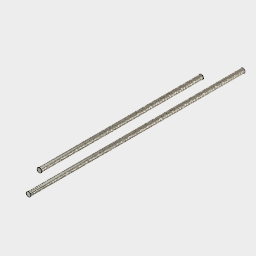
X_Axis_v8 (Autodesk Fusion 360 archive; units mm, degrees)
design "Z Linear Rods"
Autodesk Fusion 360 part; units mm, degrees
note: some values were not read from the file. Chosen so that the rebuilt part matches the saved one: how an offset face is resized.
sketch "Sketch1" plane through (0, 0, 0) normal (0, 1, 0) x (1, 0, 0) in component "X Linear Rods"
  circle A0 centre (0, 0) radius 3
  dimension "d1" = 6
  measures "d1" diameter of A0
extrude "Extrude1" add sketch "Sketch1" along normal mid plane 210 makes body 1 in component "Short"
extrude "Extrude1'" add sketch "Sketch1" along normal mid plane 278 separate body makes body 2 in component "Long"
component "X Linear Rods" placed x (1, 0, 0) y (0, 1, 0) z (0, 0, 1) at (0, 0, 0)
component "Short" placed x (1, 0, 0) y (0, 1, 0) z (0, 0, 1) at (-20, 0, 0) in component "X Linear Rods"
component "Long" placed x (1, 0, 0) y (0, 1, 0) z (0, 0, 1) at (0, 0, 0) in component "X Linear Rods"

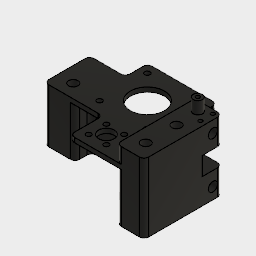
design "Z Carriage"
Autodesk Fusion 360 part; units mm, degrees
sketch "Base" plane through (0, 0, 0) normal (0, 0, 1) x (1, 0, 0) in component "Z Carriage"
  line L0 (-43.6, -8.8) -> (-23.6, -8.8)
  line L1 (-23.6, -8.8) -> (-23.6, 20.7)
  line L2 (-23.6, 20.7) -> (-43.6, 20.7)
  line L3 (-43.6, 20.7) -> (-43.6, -8.8)
  line L4 (-23.6, 2) -> (24.6, 2)
  line L5 (24.6, 2) -> (24.6, 5.65)
  line L6 (24.6, 5.65) -> (-23.6, 5.65)
  line L7 (-23.6, 5.65) -> (-23.6, 2)
  line L8 (24.6, 20.7) -> (42.4, 20.7)
  line L9 (42.4, 20.7) -> (42.4, -30)
  line L10 (42.4, -30) -> (24.6, -30)
  line L11 (24.6, -30) -> (24.6, 20.7)
  line L12 (35.44, 20.7) -> (35.44, 14.8) construction
  line L13 (38.78, 20.7) -> (38.78, 18.14)
  line L14 (32.1, 20.7) -> (32.1, 18.14)
  line L15 (32.1, 18.14) -> (38.78, 18.14) construction
  arc A0 (32.1, 18.14) -> (38.78, 18.14) centre (35.44, 18.14) ccw
  circle A1 centre (35.44, 18.14) radius 1.25
  circle A2 centre (-33.5, 0) radius 6
  circle A3 centre (-33.5, 0) radius 3
  circle A4 centre (33.5, 0) radius 3
  circle A5 centre (33.5, 0) radius 6
  circle A6 centre (33.5, -20) radius 6
  circle A7 centre (33.5, -20) radius 3
  line L16 (33.5, -20) -> (33.5, 0) construction
  line L17 (33.5, 0) -> (-33.5, 0) construction
  line L18 (33.5, -30) -> (33.5, -20) construction
  point P0 (35.44, 18.14)
  point P1 (33.5, -26)
  dimension "d1" = 48.2
  dimension "d2" = 20
  dimension "d3" = 17.8
  dimension "d4" = 3.65
  dimension "d5" = 29.5
  dimension "d6" = 50.7
  dimension "d8" = 32
  dimension "d9" = 5.9
  dimension "d11" = 6.68
  dimension "d12" = 7.5
  dimension "d13" = 2.5
  dimension "d14" = 12
  dimension "d15" = 6
  dimension "d16" = 6
  dimension "d17" = 12
  dimension "d18" = 12
  dimension "d19" = 6
  dimension "d20" = 67
  dimension "d21" = 20
  dimension "d23" = 4
  measures "d1" distance of L5.end L6.end
  measures "d2" distance of L1.end L2.end
  measures "d3" distance of L8.start L8.end
  measures "d4" distance of L4 L6
  measures "d5" distance of L0.start L2.end
  measures "d6" distance of L8.end L9.end
  measures "d8" distance of L4 L10.end
  measures "d9" distance of L12.start L12.end
  measures "d11" distance of L13.start L14.start
  measures "d12" distance of L8.start L14.start
  measures "d13" diameter of A1
  measures "d14" diameter of A2
  measures "d15" diameter of A3
  measures "d16" diameter of A4
  measures "d17" diameter of A5
  measures "d18" diameter of A6
  measures "d19" diameter of A7
  measures "d20" distance of A4.centre A2.centre
  measures "d21" distance of A6.centre A4.centre
  measures "d23" distance of L18.start P1
extrude "Extrude1" add sketch "Base" along normal blind 35 contours L0 L1 L2 L3 L7 | L1 L4 L5 L6 L7 L11 | A2 in component "Z Carriage"
extrude "Extrude2" add sketch "Base" along normal blind 45 contours L5 L8 L9 L10 L11 L13 L14 A0 | L8 L13 L14 A0 | A1 | A5 | A6 in component "Z Carriage"
extrude "Extrude3" add sketch "Base" against normal blind 3 contours L8 L13 L14 A0 in component "Z Carriage"
fillet "Fillet1" radius 3 12 edges at (24.6, 2, 17.5) (24.6, 5.65, 17.5) (-23.6, 2, 17.5) (-23.6, 5.65, 17.5) (-23.6, 20.7, 17.5) (-43.6, 20.7, 17.5) (-43.6, -8.8, 17.5) (-23.6, -8.8, 17.5) (24.6, 20.7, 22.5) (42.4, 20.7, 22.5) (42.4, -30, 22.5) (24.6, -30, 22.5) in component "Z Carriage"
sketch "Top Endstop Mount" plane through (0, 0, 35) normal (0, 0, 1) x (-1, 0, 0) in component "Z Carriage"
  line L0 (26.6, -20.7) -> (20.4, -20.7)
  line L1 (20.4, -20.7) -> (20.4, -35.1993)
  line L2 (20.4, -35.1993) -> (-24.6, -35.1993)
  line L3 (-24.6, -35.1993) -> (-24.6, -17.7)
  line L4 (-27.6, 30) -> (-39.4, 30)
  line L5 (26.6, -20.7) -> (40.6, -20.7)
  arc A0 (40.6, -20.7) -> (43.6, -17.7) centre (40.6, -17.7) ccw
  line L6 (43.6, -17.7) -> (43.6, 5.8)
  arc A1 (43.6, 5.8) -> (40.6, 8.8) centre (40.6, 5.8) ccw
  line L7 (40.6, 8.8) -> (26.6, 8.8)
  arc A2 (-24.6, 27) -> (-27.6, 30) centre (-27.6, 27) ccw
  line L8 (-24.6, -17.7) -> (-24.6, 27)
  line L9 (-27.6, 30) -> (5.6, 30)
  line L10 (5.6, 30) -> (5.6, 8.8)
  line L11 (5.6, 8.8) -> (26.6, 8.8)
  arc A3 (-39.4, 30) -> (-42.4, 27) centre (-39.4, 27) ccw
  line L12 (-42.4, 27) -> (-42.4, -17.7)
  arc A4 (-42.4, -17.7) -> (-39.4, -20.7) centre (-39.4, -17.7) ccw
  line L13 (-39.4, -20.7) -> (-27.6, -20.7)
  arc A5 (-27.6, -20.7) -> (-24.6, -17.7) centre (-27.6, -17.7) ccw
  line L14 (15.1, -29.6993) -> (-15.9, -29.6993) construction
  line L15 (-15.9, -29.6993) -> (-15.9, 1.3007) construction
  line L16 (-15.9, 1.3007) -> (15.1, 1.3007) construction
  line L17 (15.1, 1.3007) -> (15.1, -29.6993) construction
  line L18 (15.1, 1.3007) -> (-15.9, -29.6993) construction
  circle A6 centre (-0.4, -14.1993) radius 11
  circle A7 centre (15.1, -29.6993) radius 1.725
  circle A8 centre (-15.9, -29.6993) radius 1.725
  circle A9 centre (-15.9, 1.3007) radius 1.725
  circle A10 centre (15.1, 1.3007) radius 1.725
  line L19 (-0.25, 12.25) -> (-11.75, 12.25) construction
  line L20 (-11.75, 12.25) -> (-11.75, 23.75) construction
  line L21 (-11.75, 23.75) -> (-0.25, 23.75) construction
  line L22 (-0.25, 23.75) -> (-0.25, 12.25) construction
  circle A11 centre (-11.75, 12.25) radius 1.65
  circle A12 centre (-11.75, 23.75) radius 1.65
  circle A13 centre (-0.25, 23.75) radius 1.65
  circle A14 centre (-0.25, 12.25) radius 1.65
  line L23 (-0.25, 23.75) -> (-11.75, 12.25) construction
  circle A15 centre (-6, 18) radius 5
  line L24 (-27.6, -20.7) -> (-24.6, -20.7)
  circle A16 centre (33.5, 0) radius 3
  circle A17 centre (33.5, 0) radius 3
  circle A18 centre (-33.5, 20) radius 3
  point P0 (-24.6, -17.7)
  point P1 (20.6, -5.65)
  dimension "d31" = 48
  dimension "d32" = 45
  dimension "d33" = 29.55
  dimension "d34" = 31
  dimension "d35" = 31
  dimension "d36" = 22
  dimension "d37" = 44
  dimension "d38" = 3.45
  dimension "d39" = 3.45
  dimension "d40" = 3.45
  dimension "d41" = 3.45
  dimension "d42" = 21
  dimension "d43" = 11.5
  dimension "d44" = 11.5
  dimension "d45" = 3.3
  dimension "d46" = 3.3
  dimension "d47" = 3.3
  dimension "d48" = 3.3
  dimension "d49" = 10
  dimension "d85" = 27.5
  dimension "d86" = 2
  measures "d31" distance of L9.end A3.end
  measures "d32" distance of L1.end L2.end
  measures "d33" distance of L1.end P1
  measures "d34" distance of L14.start L14.end
  measures "d35" distance of L14.start L16.end
  measures "d36" diameter of A6
  measures "d37" distance of L6 A6.centre
  measures "d38" diameter of A7
  measures "d39" diameter of A8
  measures "d40" diameter of A9
  measures "d41" diameter of A10
  measures "d42" distance of L2 A6.centre
  measures "d43" distance of L19.start L19.end
  measures "d44" distance of L19.start L21.end
  measures "d45" diameter of A11
  measures "d46" diameter of A12
  measures "d47" diameter of A13
  measures "d48" diameter of A14
  measures "d49" diameter of A15
  measures "d85" distance of A15.centre A18.centre
  measures "d86" distance of A15.centre A18.centre
extrude "Extrude4" add sketch "Top Endstop Mount" against normal blind 3 contours L0 L1 L2 L3 L5 A0 L6 A1 L7 A2 L8 L9 L10 L11 | L3 A5 L24 in component "Z Carriage"
extrude "Extrude10" cut sketch "Top Endstop Mount" against normal blind 3 contours A6 in component "Z Carriage"
extrude "Extrude7" add sketch "Top Endstop Mount" along normal blind 10 contours L3 A5 L24 in component "Z Carriage"
fillet "Fillet2" radius 3 5 edges at (-20.4, 35.1993, 33.5) (-20.4, 20.7, 33.5) (-5.6, -8.8, 33.5) (-5.6, -30, 33.5) (24.6, 35.1993, 33.5) in component "Z Carriage"
sketch "Face" plane through (42.4, 0, 0) normal (1, 0, 0) x (0, 1, 0) in component "Z Carriage"
  line L0 (14.7, 37.5) -> (14.7, 7.5) construction
  circle A0 centre (14.7, 37.5) radius 3
  circle A1 centre (14.7, 7.5) radius 3
  line L1 (20.7, 0) -> (20.7, 45)
  line L2 (20.7, 22.5) -> (14.7, 22.5) construction
  line L3 (20.7, 28.4) -> (7.73, 28.4)
  line L4 (7.73, 28.4) -> (7.73, 16.6)
  line L5 (7.73, 16.6) -> (20.7, 16.6)
  point P0 (7.73, 22.5)
  dimension "d55" = 6
  dimension "d56" = 6
  dimension "d58" = 30
  dimension "d59" = 6
  dimension "d64" = 12.97
  dimension "d65" = 11.8
  measures "d55" diameter of A0
  measures "d56" diameter of A1
  measures "d58" distance of L0.start L0.end
  measures "d59" distance of L2.start L2.end
  measures "d64" distance of L3.start L3.end
  measures "d65" distance of L3.end L4.end
extrude "Extrude5" cut sketch "Face" against normal blind 17.81 contours A0 | L1 L3 L4 L5 in component "Z Carriage"
extrude "Extrude6" cut sketch "Face" against normal blind 86 contours A1 in component "Z Carriage"
sketch "Top Mount" plane through (0, 0, 45) normal (0, 0, 1) x (-1, 0, 0) in component "Z Carriage"
  arc A0 (-24.6, 27) -> (-27.6, 30) centre (-27.6, 27) ccw
  line L0 (-27.6, 30) -> (-39.4, 30)
  arc A1 (-39.4, 30) -> (-42.4, 27) centre (-39.4, 27) ccw
  line L1 (-42.4, 27) -> (-42.4, -17.7)
  arc A2 (-42.4, -17.7) -> (-39.4, -20.7) centre (-39.4, -17.7) ccw
  line L2 (-39.4, -20.7) -> (-24.6, -20.7)
  line L3 (-27.6, -20.7) -> (-24.6, -20.7)
  line L4 (-39.4, -20.7) -> (-27.6, -20.7)
  arc A3 (-42.4, -17.7) -> (-39.4, -20.7) centre (-39.4, -17.7) ccw
  line L5 (-42.4, 27) -> (-42.4, -17.7)
  arc A4 (-24.6, 27) -> (-27.6, 30) centre (-27.6, 27) ccw
  line L6 (-27.6, 30) -> (-39.4, 30)
  arc A5 (-39.4, 30) -> (-42.4, 27) centre (-39.4, 27) ccw
  line L7 (-24.6, -20.7) -> (-24.6, 27)
  circle A6 centre (-32.6, -14.7) radius 3
  circle A7 centre (-32.6, -14.7) radius 1.25
  line L8 (-38.95, -18.07) -> (-38.95, -10.07)
  circle A8 centre (-38.95, -18.07) radius 1.25
  circle A9 centre (-38.95, -10.07) radius 1.25
  circle A10 centre (-33.5, 20) radius 3
  circle A11 centre (-33.5, 0) radius 3
  circle A12 centre (-33.5, 0) radius 3
  circle A13 centre (-33.5, 20) radius 3
  dimension "d70" = 6
  dimension "d71" = 2.5
  dimension "d72" = 6
  dimension "d73" = 8
  dimension "d74" = 2.5
  dimension "d75" = 2.5
  dimension "d76" = 8
  dimension "d77" = 2.63
  dimension "d78" = 3.45
  measures "d70" diameter of A6
  measures "d71" diameter of A7
  measures "d72" distance of L2.end A6.centre
  measures "d73" distance of L2.end A6.centre
  measures "d74" diameter of A8
  measures "d75" diameter of A9
  measures "d76" distance of L8.start L8.end
  measures "d77" distance of A2.end L8.start
  measures "d78" distance of L1.end L8.start
extrude "Extrude8" add sketch "Top Mount" along normal blind 8 contours A6 in component "Z Carriage"
extrude "Extrude9" cut sketch "Top Mount" against normal blind 5 contours A8 | A9 in component "Z Carriage"
component "Z Carriage" placed x (1, 0, 0) y (0, 1, 0) z (0, 0, 1) at (0, 0, 0)
equation "d77 = 1.38 mm + d74 / 2"
equation "d78 = 2.2 mm + d74 / 2"

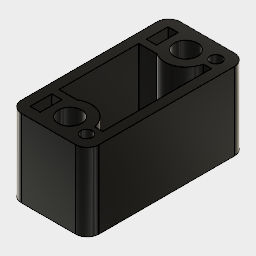
design "X End Bracket"
Autodesk Fusion 360 part; units mm, degrees
sketch "Outside" plane through (0, 0, 0) normal (0, 0, 1) x (1, 0, 0) in component "X End Bracket"
  line L0 (10, -20.5) -> (-10, -20.5)
  line L1 (-10, -20.5) -> (-10, 20.5)
  line L2 (-10, 20.5) -> (10, 20.5)
  line L3 (10, 20.5) -> (10, -20.5)
  line L4 (0, -20.5) -> (0, 20.5) construction
  circle A0 centre (0, 0) radius 2.95
  circle A1 centre (0, 0) radius 1.6
  circle A2 centre (0, 14.965) radius 3
  circle A3 centre (0, 14.965) radius 1.575
  line L5 (10, 0) -> (-10, 0) construction
  line L6 (6, 16.7) -> (6, -16.7)
  circle A4 centre (6, 16.7) radius 1.5
  circle A5 centre (6, -16.7) radius 1.5
  circle A6 centre (0, -14.965) radius 3
  circle A7 centre (0, -14.965) radius 1.575
  circle A8 centre (0, 0) radius 5
  point P0 (6, 0)
  dimension "d1" = 20
  dimension "d2" = 41
  dimension "d3" = 5.9
  dimension "d4" = 3.2
  dimension "d5" = 6
  dimension "d6" = 3.15
  dimension "d8" = 14.965
  dimension "d9" = 3
  dimension "d10" = 3
  dimension "d11" = 33.4
  dimension "d12" = 4
  dimension "d32" = 10
  measures "d1" distance of L0.start L0.end
  measures "d2" distance of L0.start L2.end
  measures "d3" diameter of A0
  measures "d4" diameter of A1
  measures "d5" diameter of A2
  measures "d6" diameter of A3
  measures "d8" distance of A2.centre L5.end
  measures "d9" diameter of A4
  measures "d10" diameter of A5
  measures "d11" distance of L6.start L6.end
  measures "d12" distance of L3 L6
  measures "d32" diameter of A8
extrude "Extrude1" add sketch "Outside" along normal blind 20 contours L0 L1 L2 L3 | A0 | A8 in component "X End Bracket"
extrude "Extrude2" add sketch "Outside" along normal blind 1.88 contours A2 | A6 in component "X End Bracket"
extrude "Extrude3" cut sketch "Outside" along normal blind 3 contours A0 in component "X End Bracket"
fillet "Fillet1" radius 3 4 edges at (10, 20.5, 10) (-10, 20.5, 10) (-10, -20.5, 10) (10, -20.5, 10) in component "X End Bracket"
sketch "Inside" plane through (0, 0, 20) normal (0, 0, 1) x (-1, 0, 0) in component "X End Bracket"
  circle A0 centre (0, 14.965) radius 3
  circle A1 centre (-6, -16.7) radius 1.5
  circle A2 centre (-6, 16.7) radius 1.5
  circle A3 centre (0, -14.965) radius 3 construction
  arc A4 (-7, 20.5) -> (-10, 17.5) centre (-7, 17.5) ccw
  line L0 (-10, 17.5) -> (-10, -17.5)
  arc A5 (-10, -17.5) -> (-7, -20.5) centre (-7, -17.5) ccw
  line L1 (-7, -20.5) -> (7, -20.5)
  arc A6 (7, -20.5) -> (10, -17.5) centre (7, -17.5) ccw
  line L2 (10, -17.5) -> (10, 17.5)
  arc A7 (10, 17.5) -> (7, 20.5) centre (7, 17.5) ccw
  line L3 (7, 20.5) -> (-7, 20.5)
  line L4 (-10, 0) -> (10, 0) construction
  line L5 (0, -20.5) -> (0, 20.5) construction
  line L6 (-10, 17.5) -> (-10, -17.5)
  arc A8 (-10, -17.5) -> (-7, -20.5) centre (-7, -17.5) ccw
  line L7 (-7, -20.5) -> (7, -20.5)
  arc A9 (7, -20.5) -> (10, -17.5) centre (7, -17.5) ccw
  line L8 (10, -17.5) -> (10, 17.5)
  arc A10 (10, 17.5) -> (7, 20.5) centre (7, 17.5) ccw
  line L9 (7, 20.5) -> (-7, 20.5)
  arc A11 (-7, 20.5) -> (-10, 17.5) centre (-7, 17.5) ccw
  line L10 (-10, -17.5) -> (-10, 17.5)
  circle A12 centre (-6, -16.7) radius 1.5
  circle A13 centre (0, -14.965) radius 3
  circle A14 centre (0, 14.965) radius 3
  circle A15 centre (-6, 16.7) radius 1.5
  circle A16 centre (0, -14.965) radius 5.5 construction
  line L11 (10, -10.3) -> (2.9134, -10.3)
  line L12 (-10, -14) -> (-5.4147, -14)
  line L13 (7.45, -17.8) -> (4.85, -17.8)
  line L14 (4.85, -17.8) -> (4.85, -12.2)
  line L15 (4.85, -12.2) -> (7.45, -12.2)
  line L16 (7.45, -12.2) -> (7.45, -17.8)
  arc A17 (2.9134, -10.3) -> (-5.4147, -14) centre (0, -14.965) ccw
  line L17 (4.85, 17.8) -> (4.85, 12.2)
  line L18 (4.85, 12.2) -> (7.45, 12.2)
  line L19 (7.45, 17.8) -> (4.85, 17.8)
  line L20 (7.45, 12.2) -> (7.45, 17.8)
  line L21 (10, 10.3) -> (2.9134, 10.3)
  arc A18 (-5.4147, 14) -> (2.9134, 10.3) centre (0, 14.965) ccw
  line L22 (-10, 14) -> (-5.4147, 14)
  line L23 (7.5, -10.3) -> (7.5, 10.3)
  line L24 (-7.5, -14) -> (-7.5, 14)
  dimension "d20" = 11
  dimension "d22" = 10.3
  dimension "d23" = 14
  dimension "d24" = 5.6
  dimension "d25" = 1.9
  dimension "d26" = 2.55
  dimension "d27" = 2.6
  dimension "d28" = 2.5
  dimension "d29" = 2.5
  measures "d20" diameter of A16
  measures "d22" distance of L4.end L11
  measures "d23" distance of L4.start L12
  measures "d24" distance of L13.start L15.end
  measures "d25" distance of L11.start L15.end
  measures "d26" distance of A6.end L13.start
  measures "d27" distance of L13.start L13.end
  measures "d28" distance of L2 L23
  measures "d29" distance of L0 L24
extrude "Extrude4" cut sketch "Inside" against normal blind 17 contours L11 L12 A17 L21 A18 L22 L23 L24 | L13 L14 L15 L16 | L17 L18 L19 L20 in component "X End Bracket"
extrude "Extrude5" add sketch "Outside" along normal blind 1.5 from surface at 3 contours A0 | A8 in component "X End Bracket"
component "X End Bracket" placed x (1, 0, 0) y (0, 1, 0) z (0, 0, 1) at (0, 0, 0)
equation "d8 = ( 29.93 / 2 ) * 1 mm"
equation "d22 = ( 20.6 / 2 ) * 1 mm"
equation "d23 = ( 28 / 2 ) * 1 mm"

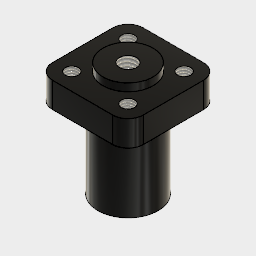
design "Lead Srew Nut"
Autodesk Fusion 360 part; units mm, degrees
sketch "Sketch1" plane through (0, 0, 0) normal (0, 0, 1) x (1, 0, 0) in component "Lead Srew Nut"
  circle A0 centre (0, 0) radius 4.9
  circle A1 centre (0, 0) radius 5.9
  circle A2 centre (0, 0) radius 2
  line L0 (-5.9, 8.9) -> (5.9, 8.9)
  line L1 (8.9, 5.9) -> (8.9, -5.9)
  line L2 (5.9, -8.9) -> (-5.9, -8.9)
  line L3 (-8.9, -5.9) -> (-8.9, 5.9)
  line L4 (-8.9, 8.9) -> (8.9, -8.9) construction
  line L5 (8.9, 8.9) -> (-8.9, -8.9) construction
  circle A3 centre (-5.5, 5.5) radius 1.5
  circle A4 centre (-5.5, -5.5) radius 1.5
  circle A5 centre (5.5, -5.5) radius 1.5
  circle A6 centre (5.5, 5.5) radius 1.5
  arc A7 (-5.9, 8.9) -> (-8.9, 5.9) centre (-5.9, 5.9) ccw
  arc A8 (8.9, 5.9) -> (5.9, 8.9) centre (5.9, 5.9) ccw
  arc A9 (5.9, -8.9) -> (8.9, -5.9) centre (5.9, -5.9) ccw
  arc A10 (-8.9, -5.9) -> (-5.9, -8.9) centre (-5.9, -5.9) ccw
  dimension "d1" = 9.8
  dimension "d2" = 11.8
  dimension "d3" = 4
  dimension "d4" = 17.8
  dimension "d5" = 17.8
  dimension "d6" = 3
  dimension "d7" = 5.5
  dimension "d9" = 360
  dimension "d10" = 3
  measures "d1" diameter of A0
  measures "d2" diameter of A1
  measures "d3" diameter of A2
  measures "d4" distance of L5.start L4.end
  measures "d5" distance of L4.start L5.start
  measures "d6" diameter of A3
  measures "d7" distance of A0.centre A3.centre
  measures "d10" radius of A7
extrude "Extrude1" add sketch "Sketch1" along normal blind 5 contours A0 | A1 | L0 L1 L2 L3 A7 A8 A9 A10 in component "Lead Srew Nut"
extrude "Extrude2" add sketch "Sketch1" along normal blind 1.5 from surface at 5 contours A0 in component "Lead Srew Nut"
extrude "Extrude3" add sketch "Sketch1" against normal blind 15.7 contours A0 | A1 in component "Lead Srew Nut"
thread "Thread1" "ISO Metric profile 4.0 M4x0.7 6H" major diameter 4.1095 minor diameter 3.332 pitch 0.7 angle 60 resizes the face on face at (1.9901, -0.1991, 4.3333) in component "Lead Srew Nut"
thread "Thread2" "ISO Metric profile 3.0 M3x0.5 6H" major diameter 3.086 minor diameter 2.529 pitch 0.5 angle 60 resizes the face on face at (6.9981, 5.5748, 1.6667) on face at (-4.0019, 5.5748, 1.6667) on face at (-4.0019, -5.4252, 1.6667) on face at (6.9981, -5.4252, 1.6667) in component "Lead Srew Nut"
component "Lead Srew Nut" placed x (1, 0, 0) y (0, 1, 0) z (0, 0, 1) at (0, 0, 0)
equation "d7 = ( 11 / 2 ) * 1 mm"
